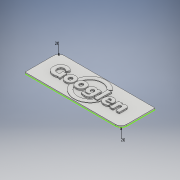
# Autodesk Inventor part: Googlen
Saved by Autodesk Inventor 2017 (Build 210142000, 142)
## iProperties
Created: 2019-03-06
Part Number: Googlen
Material: Generic
Document SubType Name: Modeling
Designer: Daniel Serena
Density: 1 g/cm^3
Appearance: Default
Author: Daniel Serena
Autodesk Inventor part; units mm, degrees
ref_plane "YZ Plane" through (0, 0, 0) normal (1, 0, 0) x (0, 1, 0)
ref_plane "XZ Plane" through (0, 0, 0) normal (0, 1, 0) x (-1, 0, 0)
ref_plane "XY Plane" through (0, 0, 0) normal (0, 0, 1) x (1, 0, 0)
sketch "Sketch1" plane through (0, 0, 0) normal (0, 0, 1) x (1, 0, 0)
  line L0 (-91.6033, 98.5763) -> (1273.941, 98.5763) construction
  line L1 (1273.941, 98.5763) -> (1273.941, -107.5318) construction
  line L2 (1273.941, -107.5318) -> (-91.6033, -107.5318) construction
  line L3 (-91.6033, -107.5318) -> (-91.6033, 98.5763) construction
  line L4 (-127.5194, 10.0678) -> (192.919, 10.0678)
  line L5 (212.919, 30.0678) -> (212.919, 130.2819)
  line L6 (212.919, 130.2819) -> (-107.5194, 130.2819)
  line L7 (-127.5194, 110.2819) -> (-127.5194, 10.0678)
  line L8 (-127.5194, 10.0678) -> (212.919, 130.2819) construction
  line L9 (212.919, 10.0678) -> (-127.5194, 130.2819) construction
  arc A0 (-107.5194, 130.2819) -> (-127.5194, 110.2819) centre (-107.5194, 110.2819) ccw
  arc A1 (192.919, 10.0678) -> (212.919, 30.0678) centre (192.919, 30.0678) ccw
  arc A2 (85.5039, 107.3952) -> (99.4232, 70.1749) centre (42.6998, 70.1749) ccw
  arc A3 (74.7241, 98.5763) -> (83.0614, 55.9225) centre (42.6998, 70.1749) ccw
  line L10 (42.6998, 70.1749) -> (99.4232, 70.1749)
  line L11 (42.6998, 70.1749) -> (42.6998, 55.5191)
  line L12 (42.6998, 55.5191) -> (82.9167, 55.5191)
  line L13 (74.7241, 98.5763) -> (85.5039, 107.3952)
  spline S0 degree 2 poles (-42.5038, 49.5943) (-42.4255, 48.6546) (-43.4827, 48.6546) knots 0 0 0 1 1 1
  spline S1 degree 2 poles (-43.4827, 48.6546) (-44.1483, 48.6546) (-50.4521, 50.1816) (-51.196, 50.4557) knots 0 0 0 1 2 2 2
  spline S2 degree 2 poles (-51.196, 50.4557) (-58.4787, 47.6366) (-65.1741, 47.6366) knots 0 0 0 1 1 1
  spline S3 degree 2 poles (-65.1741, 47.6366) (-75.9415, 47.6366) (-82.8327, 54.8018) knots 0 0 0 1 1 1
  spline S4 degree 2 poles (-82.8327, 54.8018) (-89.6847, 61.8887) (-89.6847, 72.6953) knots 0 0 0 1 1 1
  spline S5 degree 2 poles (-89.6847, 72.6953) (-89.6847, 83.7759) (-83.0676, 91.0586) knots 0 0 0 1 1 1
  spline S6 degree 2 poles (-83.0676, 91.0586) (-76.2156, 98.5763) (-65.2916, 98.5763) knots 0 0 0 1 1 1
  spline S7 degree 2 poles (-65.2916, 98.5763) (-60.0058, 98.5763) (-55.3072, 96.5402) knots 0 0 0 1 1 1
  spline S8 degree 2 poles (-55.3072, 96.5402) (-50.2563, 94.3084) (-47.3589, 90.2756) knots 0 0 0 1 1 1
  spline S9 degree 2 poles (-47.3589, 90.2756) (-46.7716, 89.4533) (-46.7716, 89.1009) knots 0 0 0 1 1 1
  spline S10 degree 2 poles (-46.7716, 89.1009) (-46.7716, 87.9655) (-52.9971, 80.2129) (-53.8977, 80.2129) knots 0 0 0 1 2 2 2
  spline S11 degree 2 poles (-53.8977, 80.2129) (-54.1326, 80.2129) (-55.5422, 81.6225) knots 0 0 0 1 1 1
  spline S12 degree 2 poles (-55.5422, 81.6225) (-57.2258, 83.3452) (-59.0269, 84.2849) knots 0 0 0 1 1 1
  spline S13 degree 2 poles (-59.0269, 84.2849) (-61.6894, 85.6945) (-64.9, 85.6945) knots 0 0 0 1 1 1
  spline S14 degree 2 poles (-64.9, 85.6945) (-70.1076, 85.6945) (-73.2007, 81.7791) knots 0 0 0 1 1 1
  spline S15 degree 2 poles (-73.2007, 81.7791) (-76.059, 78.216) (-76.059, 72.8519) knots 0 0 0 1 1 1
  spline S16 degree 2 poles (-76.059, 72.8519) (-76.059, 67.1745) (-73.0833, 63.8464) knots 0 0 0 1 1 1
  spline S17 degree 2 poles (-73.0833, 63.8464) (-70.0292, 60.44) (-64.391, 60.44) knots 0 0 0 1 1 1
  spline S18 degree 2 poles (-64.391, 60.44) (-60.828, 60.44) (-56.4427, 62.2019) knots 0 0 0 1 1 1
  spline S19 degree 2 poles (-56.4427, 62.2019) (-56.5602, 63.3766) (-57.0692, 68.0751) knots 0 0 0 1 1 1
  spline S20 degree 2 poles (-57.0692, 68.0751) (-57.539, 71.7164) (-57.539, 73.9482) knots 0 0 0 1 1 1
  spline S21 degree 2 poles (-57.539, 73.9482) (-57.539, 74.5747) (-57.0692, 74.7313) knots 0 0 0 1 1 1
  spline S22 degree 2 poles (-57.0692, 74.7313) (-56.9126, 74.8096) (-56.521, 74.8096) knots 0 0 0 1 1 1
  spline S23 degree 2 poles (-56.521, 74.8096) (-55.503, 74.8096) (-51.431, 74.4181) (-50.3738, 74.4181) knots 0 0 0 1 2 2 2
  spline S24 degree 2 poles (-50.3738, 74.4181) (-49.2775, 74.4181) (-44.8139, 74.7313) (-43.6784, 74.7313) knots 0 0 0 1 2 2 2
  spline S25 degree 2 poles (-43.6784, 74.7313) (-42.817, 74.7313) (-42.817, 73.5958) knots 0 0 0 1 1 1
  spline S26 degree 2 poles (-42.817, 73.5958) (-42.817, 71.9122) (-43.2086, 65.1385) (-43.2086, 63.4549) knots 0 0 0 1 2 2 2
  spline S27 degree 2 poles (-43.2086, 63.4549) (-43.2086, 58.9521) (-42.543, 49.9858) knots 0 0 0 1 1 1
  line L14 (-42.543, 49.9858) -> (-42.5038, 49.5943)
  spline S28 degree 2 poles (-4.2892, 65.6475) (-4.2892, 57.6992) (-14.0386, 47.7932) (-21.9478, 47.7932) knots 0 0 0 1 2 2 2
  spline S29 degree 2 poles (-21.9478, 47.7932) (-29.622, 47.7932) (-39.5281, 57.5817) (-39.5281, 65.256) knots 0 0 0 1 2 2 2
  spline S30 degree 2 poles (-39.5281, 65.256) (-39.5281, 73.3218) (-30.0527, 83.4236) (-21.9478, 83.4236) knots 0 0 0 1 2 2 2
  spline S31 degree 2 poles (-21.9478, 83.4236) (-14.0386, 83.4236) (-4.2892, 73.5567) (-4.2892, 65.6475) knots 0 0 0 1 2 2 2
  spline S32 degree 2 poles (-15.7223, 65.6475) (-15.7223, 68.4275) (-19.1287, 72.6561) (-21.8695, 72.6561) knots 0 0 0 1 2 2 2
  spline S33 degree 2 poles (-21.8695, 72.6561) (-24.6495, 72.6561) (-26.4114, 70.5026) knots 0 0 0 1 1 1
  spline S34 degree 2 poles (-26.4114, 70.5026) (-28.095, 68.4666) (-28.095, 65.6475) knots 0 0 0 1 1 1
  spline S35 degree 2 poles (-28.095, 65.6475) (-28.095, 62.8284) (-26.4114, 60.7924) knots 0 0 0 1 1 1
  spline S36 degree 2 poles (-26.4114, 60.7924) (-24.6495, 58.6389) (-21.8695, 58.6389) knots 0 0 0 1 1 1
  spline S37 degree 2 poles (-21.8695, 58.6389) (-19.1287, 58.6389) (-17.3668, 60.7924) knots 0 0 0 1 1 1
  spline S38 degree 2 poles (-17.3668, 60.7924) (-15.7223, 62.8284) (-15.7223, 65.6475) knots 0 0 0 1 1 1
  spline S39 degree 2 poles (33.4946, 65.6475) (33.4946, 57.6992) (23.7452, 47.7932) (15.8361, 47.7932) knots 0 0 0 1 2 2 2
  spline S40 degree 2 poles (15.8361, 47.7932) (8.1618, 47.7932) (-1.7442, 57.5817) (-1.7442, 65.256) knots 0 0 0 1 2 2 2
  spline S41 degree 2 poles (-1.7442, 65.256) (-1.7442, 73.3218) (7.7311, 83.4236) (15.8361, 83.4236) knots 0 0 0 1 2 2 2
  spline S42 degree 2 poles (15.8361, 83.4236) (23.7452, 83.4236) (33.4946, 73.5567) (33.4946, 65.6475) knots 0 0 0 1 2 2 2
  spline S43 degree 2 poles (22.0616, 65.6475) (22.0616, 68.4275) (18.6552, 72.6561) (15.9144, 72.6561) knots 0 0 0 1 2 2 2
  spline S44 degree 2 poles (15.9144, 72.6561) (13.1344, 72.6561) (11.3725, 70.5026) knots 0 0 0 1 1 1
  spline S45 degree 2 poles (11.3725, 70.5026) (9.6888, 68.4666) (9.6888, 65.6475) knots 0 0 0 1 1 1
  spline S46 degree 2 poles (9.6888, 65.6475) (9.6888, 62.8284) (11.3725, 60.7924) knots 0 0 0 1 1 1
  spline S47 degree 2 poles (11.3725, 60.7924) (13.1344, 58.6389) (15.9144, 58.6389) knots 0 0 0 1 1 1
  spline S48 degree 2 poles (15.9144, 58.6389) (18.6552, 58.6389) (20.4171, 60.7924) knots 0 0 0 1 1 1
  spline S49 degree 2 poles (20.4171, 60.7924) (22.0616, 62.8284) (22.0616, 65.6475) knots 0 0 0 1 1 1
  spline S50 degree 2 poles (72.4531, 57.5817) (72.4531, 47.6366) (68.2636, 43.2904) knots 0 0 0 1 1 1
  spline S51 degree 2 poles (68.2636, 43.2904) (63.9175, 38.866) (53.894, 38.866) knots 0 0 0 1 1 1
  spline S52 degree 2 poles (53.894, 38.866) (50.9574, 38.866) (45.9065, 39.8057) knots 0 0 0 1 1 1
  spline S53 degree 2 poles (45.9065, 39.8057) (39.4461, 40.9803) (39.4461, 42.5857) knots 0 0 0 1 1 1
  spline S54 degree 2 poles (39.4461, 42.5857) (39.4461, 43.2513) (40.9339, 49.4377) knots 0 0 0 1 1 1
  spline S55 degree 2 poles (40.9339, 49.4377) (41.208, 50.4165) (41.717, 50.4165) knots 0 0 0 1 1 1
  spline S56 degree 2 poles (41.717, 50.4165) (41.8736, 50.3774) (42.1086, 50.2599) knots 0 0 0 1 1 1
  spline S57 degree 2 poles (42.1086, 50.2599) (47.4727, 47.6366) (52.0538, 47.6366) knots 0 0 0 1 1 1
  spline S58 degree 2 poles (52.0538, 47.6366) (54.5596, 47.6366) (57.0264, 48.8895) knots 0 0 0 1 1 1
  spline S59 degree 2 poles (57.0264, 48.8895) (60.0412, 50.3774) (60.0412, 52.6483) knots 0 0 0 1 1 1
  line L15 (60.0412, 52.6483) -> (60.0412, 54.9976)
  spline S60 degree 2 poles (60.0412, 54.9976) (56.4782, 51.6303) (50.9183, 51.6303) knots 0 0 0 1 1 1
  spline S61 degree 2 poles (50.9183, 51.6303) (44.3404, 51.6303) (40.1117, 56.3288) knots 0 0 0 1 1 1
  spline S62 degree 2 poles (40.1117, 56.3288) (36.0397, 60.8707) (36.0397, 67.4878) knots 0 0 0 1 1 1
  spline S63 degree 2 poles (36.0397, 67.4878) (36.0397, 74.144) (39.9551, 78.5293) knots 0 0 0 1 1 1
  spline S64 degree 2 poles (39.9551, 78.5293) (44.0271, 83.1103) (50.6442, 83.1103) knots 0 0 0 1 1 1
  spline S65 degree 2 poles (50.6442, 83.1103) (55.8909, 83.1103) (58.6708, 79.3515) knots 0 0 0 1 1 1
  spline S66 degree 2 poles (58.6708, 79.3515) (59.2581, 78.5684) (59.4539, 78.5684) knots 0 0 0 1 1 1
  spline S67 degree 2 poles (59.4539, 78.5684) (59.7671, 78.5684) (59.7671, 79.8214) knots 0 0 0 1 1 1
  spline S68 degree 2 poles (59.7671, 79.8214) (59.7671, 82.6405) (60.3936, 82.6405) knots 0 0 0 1 1 1
  spline S69 degree 2 poles (60.3936, 82.6405) (60.9418, 82.6405) (71.905, 81.505) (72.1007, 81.4267) knots 0 0 0 1 2 2 2
  spline S70 degree 2 poles (72.1007, 81.4267) (72.6881, 81.2309) (72.6881, 80.5261) knots 0 0 0 1 1 1
  spline S71 degree 2 poles (72.6881, 80.5261) (72.6881, 78.0986) (72.3748, 68.5449) (72.3748, 66.1565) knots 0 0 0 1 2 2 2
  spline S72 degree 2 poles (72.3748, 66.1565) (72.3748, 64.7078) (72.4531, 58.9913) (72.4531, 57.5817) knots 0 0 0 1 2 2 2
  spline S73 degree 2 poles (60.3936, 67.2137) (60.3936, 69.7587) (57.0264, 73.4784) (54.4813, 73.4784) knots 0 0 0 1 2 2 2
  spline S74 degree 2 poles (54.4813, 73.4784) (51.8971, 73.4784) (48.5299, 69.6804) (48.5299, 67.1354) knots 0 0 0 1 2 2 2
  spline S75 degree 2 poles (48.5299, 67.1354) (48.5299, 64.5904) (51.9754, 60.9099) (54.4813, 60.9099) knots 0 0 0 1 2 2 2
  spline S76 degree 2 poles (54.4813, 60.9099) (57.0264, 60.9099) (60.3936, 64.6687) (60.3936, 67.2137) knots 0 0 0 1 2 2 2
  spline S77 degree 2 poles (91.1689, 69.4846) (91.1689, 59.9701) (91.2472, 54.8801) knots 0 0 0 1 1 1
  spline S78 degree 2 poles (91.2472, 54.8801) (91.2472, 54.0579) (91.3255, 52.1393) knots 0 0 0 1 1 1
  spline S79 degree 2 poles (91.3255, 52.1393) (91.443, 50.3382) (91.443, 49.3593) knots 0 0 0 1 1 1
  spline S80 degree 2 poles (91.443, 49.3593) (91.443, 48.6546) (90.5816, 48.4979) knots 0 0 0 1 1 1
  spline S81 degree 2 poles (90.5816, 48.4979) (89.0154, 48.2239) (84.9433, 48.2239) knots 0 0 0 1 1 1
  spline S82 degree 2 poles (84.9433, 48.2239) (80.7538, 48.2239) (79.5792, 48.4979) knots 0 0 0 1 1 1
  spline S83 degree 2 poles (79.5792, 48.4979) (78.8353, 48.6546) (78.7178, 49.4377) knots 0 0 0 1 1 1
  spline S84 degree 2 poles (78.7178, 49.4377) (78.7178, 49.5551) (78.7178, 50.9255) knots 0 0 0 1 1 1
  spline S85 degree 2 poles (78.7178, 50.9255) (78.7178, 54.0579) (78.8744, 66.4306) (78.8744, 69.4846) knots 0 0 0 1 2 2 2
  spline S86 degree 2 poles (78.8744, 69.4846) (78.8744, 84.1283) (78.9136, 82.8362) knots 0 0 0 1 1 1
  spline S87 degree 2 poles (78.9136, 82.8362) (78.7961, 90.5496) (78.0522, 96.1095) knots 0 0 0 1 1 1
  spline S88 degree 2 poles (78.0522, 96.1095) (77.9739, 96.5011) (77.9739, 96.6969) knots 0 0 0 1 1 1
  spline S89 degree 2 poles (77.9739, 96.6969) (77.9739, 97.4799) (78.8744, 97.4799) knots 0 0 0 1 1 1
  line L16 (78.8744, 97.4799) -> (91.3255, 97.4799)
  spline S90 degree 2 poles (91.3255, 97.4799) (92.1869, 97.4799) (92.1086, 96.736) knots 0 0 0 1 1 1
  line L17 (92.1086, 96.736) -> (92.0694, 96.1095)
  spline S91 degree 2 poles (92.0694, 96.1095) (91.1689, 81.0743) (91.1689, 69.4846) knots 0 0 0 1 1 1
  spline S92 degree 2 poles (129.5009, 67.4095) (129.5009, 63.8856) (127.23, 63.4157) knots 0 0 0 1 1 1
  spline S93 degree 2 poles (127.23, 63.4157) (126.8384, 63.3374) (120.0256, 62.6326) knots 0 0 0 1 1 1
  spline S94 degree 2 poles (120.0256, 62.6326) (115.9144, 62.2019) (107.7311, 61.5755) knots 0 0 0 1 1 1
  spline S95 degree 2 poles (107.7311, 61.5755) (108.201, 59.3045) (110.7069, 58.1299) knots 0 0 0 1 1 1
  spline S96 degree 2 poles (110.7069, 58.1299) (112.7037, 57.151) (115.2879, 57.151) knots 0 0 0 1 1 1
  spline S97 degree 2 poles (115.2879, 57.151) (118.3811, 57.151) (121.5134, 58.8347) knots 0 0 0 1 1 1
  spline S98 degree 2 poles (121.5134, 58.8347) (122.8447, 59.6569) (124.1759, 60.4792) knots 0 0 0 1 1 1
  spline S99 degree 2 poles (124.1759, 60.4792) (124.9199, 60.1268) (128.3654, 53.7055) (128.3654, 52.8441) knots 0 0 0 1 2 2 2
  spline S100 degree 2 poles (128.3654, 52.8441) (128.3654, 52.6091) (127.8564, 52.061) knots 0 0 0 1 1 1
  spline S101 degree 2 poles (127.8564, 52.061) (123.5886, 47.4799) (114.6223, 47.4799) knots 0 0 0 1 1 1
  spline S102 degree 2 poles (114.6223, 47.4799) (106.3216, 47.4799) (101.2707, 52.3351) knots 0 0 0 1 1 1
  spline S103 degree 2 poles (101.2707, 52.3351) (96.024, 57.2293) (96.024, 65.4909) knots 0 0 0 1 1 1
  spline S104 degree 2 poles (96.024, 65.4909) (96.024, 73.5175) (100.6834, 78.6467) knots 0 0 0 1 1 1
  spline S105 degree 2 poles (100.6834, 78.6467) (105.4993, 83.9326) (113.4477, 83.9326) knots 0 0 0 1 1 1
  spline S106 degree 2 poles (113.4477, 83.9326) (120.143, 83.9326) (129.5009, 74.144) (129.5009, 67.4095) knots 0 0 0 1 2 2 2
  spline S107 degree 2 poles (117.2848, 69.5629) (117.2848, 71.7164) (114.2307, 75.0054) (112.0773, 75.0054) knots 0 0 0 1 2 2 2
  spline S108 degree 2 poles (112.0773, 75.0054) (109.8846, 75.0054) (108.4751, 73.1651) knots 0 0 0 1 1 1
  spline S109 degree 2 poles (108.4751, 73.1651) (107.1438, 71.4423) (107.1438, 69.1322) knots 0 0 0 1 1 1
  spline S110 degree 2 poles (107.1438, 69.1322) (107.1438, 68.1925) (108.1227, 68.1925) knots 0 0 0 1 1 1
  spline S111 degree 2 poles (108.1227, 68.1925) (110.7069, 68.1925) (116.1493, 69.0148) knots 0 0 0 1 1 1
  spline S112 degree 2 poles (116.1493, 69.0148) (117.2848, 69.1714) (117.2848, 69.5629) knots 0 0 0 1 1 1
  spline S113 degree 2 poles (167.9895, 49.516) (167.9895, 48.5763) (166.0318, 48.3022) (161.9206, 48.3022) knots 0 0 0 1 2 2 2
  spline S114 degree 2 poles (161.9206, 48.3022) (157.4962, 48.3022) (155.421, 48.7329) (155.421, 49.9467) knots 0 0 0 1 2 2 2
  spline S115 degree 2 poles (155.421, 49.9467) (155.421, 51.5911) (155.6168, 58.2082) (155.6168, 59.8527) knots 0 0 0 1 2 2 2
  spline S116 degree 2 poles (155.6168, 59.8527) (155.6168, 61.1448) (155.4602, 66.274) (155.4602, 67.5661) knots 0 0 0 1 2 2 2
  spline S117 degree 2 poles (155.4602, 67.5661) (155.4602, 72.3429) (151.349, 72.3429) knots 0 0 0 1 1 1
  spline S118 degree 2 poles (151.349, 72.3429) (149.9786, 72.3429) (148.1775, 71.1683) knots 0 0 0 1 1 1
  spline S119 degree 2 poles (148.1775, 71.1683) (146.2198, 69.837) (146.2198, 68.5449) knots 0 0 0 1 1 1
  line L18 (146.2198, 68.5449) -> (146.2198, 49.7117)
  spline S120 degree 2 poles (146.2198, 49.7117) (146.2198, 48.5763) (145.1235, 48.4588) knots 0 0 0 1 1 1
  spline S121 degree 2 poles (145.1235, 48.4588) (143.9097, 48.3022) (140.1509, 48.3022) knots 0 0 0 1 1 1
  spline S122 degree 2 poles (140.1509, 48.3022) (136.0788, 48.3022) (134.865, 48.4979) knots 0 0 0 1 1 1
  spline S123 degree 2 poles (134.865, 48.4979) (133.7687, 48.6937) (133.7687, 49.6726) knots 0 0 0 1 1 1
  spline S124 degree 2 poles (133.7687, 49.6726) (133.7687, 52.3742) (133.847, 63.3374) (133.847, 66.0782) knots 0 0 0 1 2 2 2
  spline S125 degree 2 poles (133.847, 66.0782) (133.847, 74.7705) (132.4766, 79.7039) knots 0 0 0 1 1 1
  spline S126 degree 2 poles (132.4766, 79.7039) (132.3983, 80.0171) (132.3983, 80.2129) knots 0 0 0 1 1 1
  spline S127 degree 2 poles (132.3983, 80.2129) (132.3983, 80.8002) (132.9073, 80.996) knots 0 0 0 1 1 1
  spline S128 degree 2 poles (132.9073, 80.996) (135.1391, 81.2309) (138.7805, 81.7791) knots 0 0 0 1 1 1
  spline S129 degree 2 poles (138.7805, 81.7791) (144.3404, 82.8362) (145.0451, 82.8362) knots 0 0 0 1 1 1
  spline S130 degree 2 poles (145.0451, 82.8362) (145.4367, 82.8362) (145.8282, 78.1377) (146.2198, 78.1377) knots 0 0 0 1 2 2 2
  spline S131 degree 2 poles (146.2198, 78.1377) (145.8282, 78.1377) (154.0898, 82.9929) (157.2221, 82.9929) knots 0 0 0 1 2 2 2
  spline S132 degree 2 poles (157.2221, 82.9929) (161.6466, 82.9929) (164.5831, 80.9177) knots 0 0 0 1 1 1
  spline S133 degree 2 poles (164.5831, 80.9177) (167.9112, 78.4901) (167.9112, 74.2223) knots 0 0 0 1 1 1
  line L19 (167.9112, 74.2223) -> (167.9112, 63.1025)
  spline S134 degree 2 poles (167.9112, 63.1025) (167.9112, 60.8315) (167.9895, 51.7869) (167.9895, 49.516) knots 0 0 0 1 2 2 2
  dimension "d2" = 20
  dimension "d3" = 20
  constraints: 20 end point, 9 point on circle, 6 point on line, 4 centre point, 4 tangent, 3 parallel, 2 coincident, 2 midpoint, 2 perpendicular, 1 horizontal, 1 vertical, 2 other
  measures "d2" radius of A0
  measures "d3" radius of A1
extrude "Extrusion1" add sketch "Sketch1" along normal blind 10 contours S31 S28 A2 | A2 S28 S29 S30 S31 | S41 S42 S39 S40 A3 | A3 S40 S41 | S103 S104 L10 A2 | A2 L10 S104 S105 S106 S92 S93 S94 S95 S96 S97 S98 S99 S100 S101 S102 S103 | S82 S83 S84 S85 L12 A3 | A3 L12 S85 S86 L10 S91 S77 S78 S79 S80 S81 S82 | L10 S86 S87 S88 S89 L16 S90 L17 S91 | S50 S51 S52 S53 S54 S55 S56 S57 S58 S59 L15 S60 S61 S62 S63 S64 S65 S66 S67 S68 S69 S70 S71 L10 S73 S74 L11 L12 | L12 L11 L10 S74 S75 S76 S73 S71 S72 S50 | S0 S1 S2 S3 S4 S5 S6 S7 S8 S9 S10 S11 S12 S13 S14 S15 S16 S17 S18 S19 S20 S21 S22 S23 S24 S25 S26 S27 L14 | S113 S114 S115 S116 S117 S118 S119 L18 S120 S121 S122 S123 S124 S125 S126 S127 S128 S129 S130 S131 S132 S133 L19 S134
extrude "Extrusion2" add sketch "Sketch1" along normal blind 5 contours L7 A0 L6 L5 A1 L4 | A2 S28 S29 S30 S31 | S41 S42 S39 S40 A3 | A2 L10 S104 S105 S106 S92 S93 S94 S95 S96 S97 S98 S99 S100 S101 S102 S103 | S82 S83 S84 S85 L12 A3 | L10 S86 S87 S88 S89 L16 S90 L17 S91 | S50 S51 S52 S53 S54 S55 S56 S57 S58 S59 L15 S60 S61 S62 S63 S64 S65 S66 S67 S68 S69 S70 S71 L10 S73 S74 L11 L12 | L10 S74 S73 | S0 S1 S2 S3 S4 S5 S6 S7 S8 S9 S10 S11 S12 S13 S14 S15 S16 S17 S18 S19 S20 S21 S22 S23 S24 S25 S26 S27 L14 | S38 S37 S36 S35 S34 S33 S32 | S49 S48 S47 S46 S45 S44 S43 | S112 S111 S110 S109 S108 S107 | S113 S114 S115 S116 S117 S118 S119 L18 S120 S121 S122 S123 S124 S125 S126 S127 S128 S129 S130 S131 S132 S133 L19 S134
extrude "Extrusion3" add sketch "Sketch1" along normal blind 7 contours L13 A3 S41 S40 S82 S81 S80 S79 S78 S77 S91 L10 S104 S103 A2 S28 S31 | S31 S28 A2 | A3 S40 S41 | S103 S104 L10 A2 | A3 L12 S85 S86 L10 S91 S77 S78 S79 S80 S81 S82 | L12 S50 S72 S71 L10 S86 S85 | L12 L11 L10 S74 S75 S76 S73 S71 S72 S50 | S73 S76 S75 S74 L10
body "Solid1"
